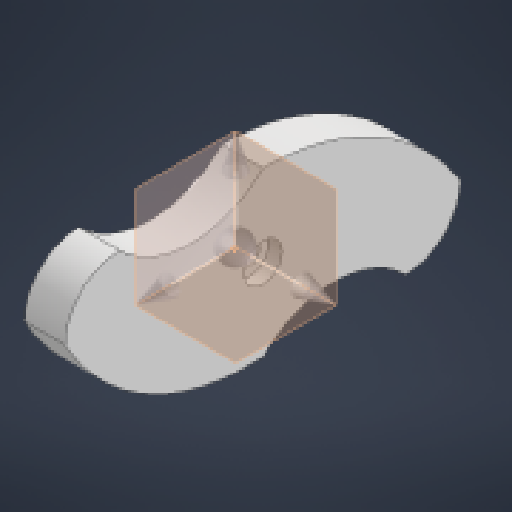
# Autodesk Inventor part: Vertical Spinner Weapon V3
Saved by Autodesk Inventor 2026.2 (Build 302298000, 298)
## iProperties
Created: 2023-08-18
Part Number: Vertical Spinner Weapon V3
Material: Generic
Document SubType Name: Modeling
Designer: vandj
Density: 1 g/cm^3
Appearance: Default
Mass: 70.3924 g
Surface Area: 175.698 cm^2
Volume: 70.3924 cm^3
Author: vandj
Autodesk Inventor part; units mm, degrees
ref_plane "YZ Plane" through (0, 0, 0) normal (1, 0, 0) x (0, 1, 0)
ref_plane "XZ Plane" through (0, 0, 0) normal (0, 1, 0) x (-1, 0, 0)
ref_plane "XY Plane" through (0, 0, 0) normal (0, 0, 1) x (1, 0, 0)
sketch "Sketch 1" plane through (0, 0, 0) normal (1, 0, 0) x (0, 1, 0)
  circle A0 centre (0, 0) radius 2.5
  circle A1 centre (0, 0) radius 25
  point P0 (1.2916, -31.2195)
  point P1 (0, 30.3272)
  point P2 (-0.1255, 30.3272)
  point P3 (0, -30.3272)
  point P4 (0.1231, -30.3272)
  point P5 (-1.2948, 31.2193)
  point P6 (0.0032, -40.9065)
  point P7 (0, -40.9065)
  point P8 (-1.4137, 30.3272)
  dimension "d22" = 5
  dimension "d51" = 50
  constraints: 2 centre point, 2 coincident
  measures "d22" diameter of A0
  measures "d51" diameter of A1
extrude "Interface" add sketch "Sketch 1" along normal blind 15
sketch "Sketch9" plane through (0, 0, 0) normal (-1, 0, 0) x (0, 0, 1)
  circle A0 centre (0, 0) radius 2.5 projected
  circle A1 centre (0, 0) radius 3.75
  dimension "d32" = 7.5
  constraints: 1 centre point, 1 coincident
  measures "d32" diameter of A1
extrude "Shaft Hole" cut sketch "Sketch9" against normal blind 28.1375
sketch "Sketch10" plane through (15, 0, 0) normal (1, 0, 0) x (0, 0, -1)
  circle A0 centre (0, 0) radius 3.75 projected
  circle A1 centre (0, 0) radius 7
  dimension "d35" = 14
  constraints: 1 centre point, 1 coincident
  measures "d35" diameter of A1
extrude "Bearing Hole" cut sketch "Sketch10" against normal blind 5
sketch "EDIT WEAPON SKETCH" plane through (0, 0, 0) normal (1, 0, 0) x (0, 1, 0)
  circle A0 centre (0, 0) radius 25 projected
  circle A1 centre (0, 0) radius 25 projected
  line L0 (83.5575, 140.0168) -> (83.5575, 44.1301) construction
  line L1 (83.5575, 44.1301) -> (66.7631, 44.1301) construction
  line L2 (66.7631, 44.1301) -> (66.7631, 140.0168) construction
  line L3 (66.7631, 140.0168) -> (83.5575, 140.0168) construction
  line L4 (-30.0586, 0) -> (-30.0586, 10)
  circle A2 centre (0, 0) radius 3.75 projected
  line L5 (-30.0586, 72.5) -> (30.0586, -72.5) construction
  line L6 (30.0586, 72.5) -> (-30.0586, -72.5) construction
  arc A3 (-30.0586, -70.5) -> (-28.0586, -72.5) centre (-28.0586, -70.5) ccw
  arc A4 (-30.0586, -52.5) -> (-10.0586, -72.5) centre (-10.0586, -52.5) ccw
  arc A5 (30.0586, 52.5) -> (10.0586, 72.5) centre (10.0586, 52.5) ccw
  arc A6 (10.0586, 72.5) -> (-30.0586, 0) centre (46.4752, 5) ccw
  arc A7 (-10.0586, -72.5) -> (30.0586, 0.1529) centre (-55.7878, 0.1529) ccw
  line L7 (30.0586, 0.1529) -> (30.0586, 0)
  line L8 (30.0586, -69.9194) -> (30.0586, -72.5)
  arc A8 (-30.0586, -52.5) -> (-30.0586, 0) centre (-56.2909, -26.25) ccw
  arc A9 (30.0586, 52.5) -> (30.0586, 0) centre (56.2909, 26.25) ccw
  point P0 (-22.6575, -10.5658)
  point P1 (22.6575, 10.5658)
  point P2 (30.0584, 0.0001)
  dimension "d63" = 2
  dimension "d64" = 20
  dimension "d65" = 20
  constraints: 18 point on circle, 10 end point, 8 tangent, 7 centre point, 2 midpoint, 2 parallel, 2 point on line, 2 other
  measures "d63" radius of A3
  measures "d64" radius of A4
  measures "d65" radius of A5
extrude "EDIT WEAPON SHAPE" add sketch "EDIT WEAPON SKETCH" along normal up to surface (15 mm away) contours A0 A9 A7 A4 A8 | A0 A8 L4 A6 A5 A9
body "Solid1"
